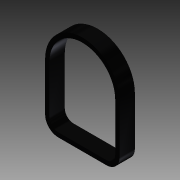
# Autodesk Inventor part: ZIP TIE EFFECTOR
Saved by Autodesk Inventor 2013 (Build 170138000, 138)
## iProperties
Created: 2014-06-22
Part Number: ZIP TIE EFFECTOR
Material: Generic
Document SubType Name: Modeling
Designer: employee
Density: 1 g/cm^3
Author: employee
Autodesk Inventor part; units mm, degrees
ref_plane "YZ Plane" through (0, 0, 0) normal (1, 0, 0) x (0, 1, 0)
ref_plane "XZ Plane" through (0, 0, 0) normal (0, 1, 0) x (-1, 0, 0)
ref_plane "XY Plane" through (0, 0, 0) normal (0, 0, 1) x (1, 0, 0)
sketch "Sketch1" plane through (0, 0, 0) normal (0, 0, 1) x (1, 0, 0)
  line L0 (1.5, -5) -> (-15, -5) construction
  line L1 (1.5, 0) -> (1.5, -5) construction
  line L2 (0, 0) -> (1.5, 0) construction
  line L3 (0, 0) -> (0, -1) construction
  arc A0 (-2, -3) -> (0, -1) centre (-2, -1) ccw construction
  line L4 (-2, -3) -> (-13, -3) construction
  arc A1 (-15, -1) -> (-13, -3) centre (-13, -1) ccw construction
  line L5 (-15, -5) -> (-15, -1) construction
  circle A2 centre (-7.5, 10) radius 7.5 construction
  line L6 (307.7386, 4.8534) -> (307.7386, -5.1466) projected
  line L7 (307.7386, -5.1466) -> (302.0236, -5.1466) projected
  line L8 (302.0236, -5.1466) -> (302.0236, 4.8534) projected
  line L9 (302.0236, 4.8534) -> (307.7386, 4.8534) projected
  circle A3 centre (304.8811, -40.1466) radius 1.5 projected
  line L10 (307.7386, -75.1466) -> (307.7386, -85.1466) projected
  line L11 (307.7386, -85.1466) -> (302.0236, -85.1466) projected
  line L12 (302.0236, -85.1466) -> (302.0236, -75.1466) projected
  line L13 (302.0236, -75.1466) -> (307.7386, -75.1466) projected
  line L14 (307.3811, 34.8534) -> (307.3811, 40.5684) projected
  line L15 (307.3811, 40.5684) -> (317.3811, 40.5684) projected
  line L16 (317.3811, 40.5684) -> (317.3811, 34.8534) projected
  line L17 (317.3811, 34.8534) -> (307.3811, 34.8534) projected
  line L18 (107.3811, 34.8534) -> (107.3811, 40.5684) projected
  line L19 (107.3811, 40.5684) -> (117.3811, 40.5684) projected
  line L20 (117.3811, 40.5684) -> (117.3811, 34.8534) projected
  line L21 (117.3811, 34.8534) -> (107.3811, 34.8534) projected
  line L22 (-92.6189, 34.8534) -> (-92.6189, 40.5684) projected
  line L23 (-92.6189, 40.5684) -> (-82.6189, 40.5684) projected
  line L24 (-82.6189, 40.5684) -> (-82.6189, 34.8534) projected
  line L25 (-82.6189, 34.8534) -> (-92.6189, 34.8534) projected
  line L26 (-128.6914, -75.1466) -> (-122.9764, -75.1466) projected
  line L27 (-122.9764, -75.1466) -> (-122.9764, -85.1466) projected
  line L28 (-122.9764, -85.1466) -> (-128.6914, -85.1466) projected
  line L29 (-128.6914, -85.1466) -> (-128.6914, -75.1466) projected
  line L30 (-57.6189, -120.8616) -> (-57.6189, -115.1466) projected
  line L31 (-57.6189, -115.1466) -> (-47.6189, -115.1466) projected
  line L32 (-47.6189, -115.1466) -> (-47.6189, -120.8616) projected
  line L33 (-47.6189, -120.8616) -> (-57.6189, -120.8616) projected
  line L34 (142.3811, -120.8616) -> (142.3811, -115.1466) projected
  line L35 (142.3811, -115.1466) -> (152.3811, -115.1466) projected
  line L36 (152.3811, -115.1466) -> (152.3811, -120.8616) projected
  line L37 (152.3811, -120.8616) -> (142.3811, -120.8616) projected
  line L38 (342.3811, -120.8616) -> (342.3811, -115.1466) projected
  line L39 (342.3811, -115.1466) -> (352.3811, -115.1466) projected
  line L40 (352.3811, -115.1466) -> (352.3811, -120.8616) projected
  line L41 (352.3811, -120.8616) -> (342.3811, -120.8616) projected
  circle A4 centre (129.8811, 37.7109) radius 1.5 projected
  circle A5 centre (-125.8339, -40.1466) radius 1.5 projected
  circle A6 centre (129.8811, -118.0041) radius 1.5 projected
  circle A7 centre (329.8811, -118.0041) radius 1.5 projected
  circle A8 centre (-70.1189, -118.0041) radius 1.5 projected
  circle A9 centre (-70.1189, 37.7109) radius 1.5 projected
  circle A10 centre (329.8811, 37.7109) radius 1.5 projected
  line L42 (307.3811, -120.8616) -> (307.3811, -115.1466) projected
  line L43 (307.3811, -115.1466) -> (317.3811, -115.1466) projected
  line L44 (317.3811, -115.1466) -> (317.3811, -120.8616) projected
  line L45 (317.3811, -120.8616) -> (307.3811, -120.8616) projected
  line L46 (107.3811, -120.8616) -> (107.3811, -115.1466) projected
  line L47 (107.3811, -115.1466) -> (117.3811, -115.1466) projected
  line L48 (117.3811, -115.1466) -> (117.3811, -120.8616) projected
  line L49 (117.3811, -120.8616) -> (107.3811, -120.8616) projected
  line L50 (-92.6189, -120.8616) -> (-92.6189, -115.1466) projected
  line L51 (-92.6189, -115.1466) -> (-82.6189, -115.1466) projected
  line L52 (-82.6189, -115.1466) -> (-82.6189, -120.8616) projected
  line L53 (-82.6189, -120.8616) -> (-92.6189, -120.8616) projected
  line L54 (-128.6914, 4.8534) -> (-122.9764, 4.8534) projected
  line L55 (-122.9764, 4.8534) -> (-122.9764, -5.1466) projected
  line L56 (-122.9764, -5.1466) -> (-128.6914, -5.1466) projected
  line L57 (-128.6914, -5.1466) -> (-128.6914, 4.8534) projected
  line L58 (-57.6189, 34.8534) -> (-57.6189, 40.5684) projected
  line L59 (-57.6189, 40.5684) -> (-47.6189, 40.5684) projected
  line L60 (-47.6189, 40.5684) -> (-47.6189, 34.8534) projected
  line L61 (-47.6189, 34.8534) -> (-57.6189, 34.8534) projected
  line L62 (142.3811, 34.8534) -> (142.3811, 40.5684) projected
  line L63 (142.3811, 40.5684) -> (152.3811, 40.5684) projected
  line L64 (152.3811, 40.5684) -> (152.3811, 34.8534) projected
  line L65 (152.3811, 34.8534) -> (142.3811, 34.8534) projected
  line L66 (342.3811, 34.8534) -> (342.3811, 40.5684) projected
  line L67 (342.3811, 40.5684) -> (352.3811, 40.5684) projected
  line L68 (352.3811, 40.5684) -> (352.3811, 34.8534) projected
  line L69 (352.3811, 34.8534) -> (342.3811, 34.8534) projected
  arc A11 (-128.6914, 43.5684) -> (-131.6914, 40.5684) centre (-128.6914, 40.5684) ccw projected
  line L70 (-131.6914, 40.5684) -> (-131.6914, -120.8616) projected
  arc A12 (-131.6914, -120.8616) -> (-128.6914, -123.8616) centre (-128.6914, -120.8616) ccw projected
  line L71 (-128.6914, -123.8616) -> (-81.6914, -123.8616) projected
  arc A13 (-26.3042, -126.9388) -> (-81.6914, -123.8616) centre (-81.6914, -623.8616) ccw projected
  line L72 (-26.3042, -126.9388) -> (277.3514, -160.7844) projected
  arc A14 (277.3514, -160.7844) -> (332.7386, -163.8616) centre (332.7386, 336.1384) ccw projected
  line L73 (332.7386, -163.8616) -> (382.7386, -163.8616) projected
  line L74 (382.7386, -163.8616) -> (382.7386, 83.5684) projected
  line L75 (382.7386, 83.5684) -> (332.7386, 83.5684) projected
  arc A15 (332.7386, 83.5684) -> (277.3514, 80.4912) centre (332.7386, -416.4316) ccw projected
  line L76 (277.3514, 80.4912) -> (-26.3042, 46.6456) projected
  arc A16 (-81.6914, 43.5684) -> (-26.3042, 46.6456) centre (-81.6914, 543.5684) ccw projected
  line L77 (-81.6914, 43.5684) -> (-128.6914, 43.5684) projected
  line L78 (0, 0) -> (0, 10)
  arc A17 (0, 10) -> (-15, 10) centre (-7.5, 10) ccw
  line L79 (-15, 10) -> (-15, -1)
  line L80 (0, 0) -> (0, -1)
  arc A18 (-2, -3) -> (0, -1) centre (-2, -1) ccw
  line L81 (-2, -3) -> (-13, -3)
  arc A19 (-15, -1) -> (-13, -3) centre (-13, -1) ccw
  line L82 (1, 10) -> (1, 0)
  line L83 (1, 0) -> (1, -1)
  arc A20 (-2, -4) -> (1, -1) centre (-2, -1) ccw
  line L84 (-2, -4) -> (-13, -4)
  arc A21 (-16, -1) -> (-13, -4) centre (-13, -1) ccw
  line L85 (-16, -1) -> (-16, 10)
  arc A22 (1, 10) -> (-16, 10) centre (-7.5, 10) ccw
  dimension "d0" = 1
  constraints: 16 end point, 14 point on circle, 11 tangent, 6 centre point, 2 collinear, 2 concentric, 2 parallel, 6 other
  measures "d0" distance between parallel lines of L82 L78
extrude "Extrusion1" add sketch "Sketch1" along normal blind 3.5 contours L82 L83 A20 L84 A21 L85 A22
body "Solid1"
